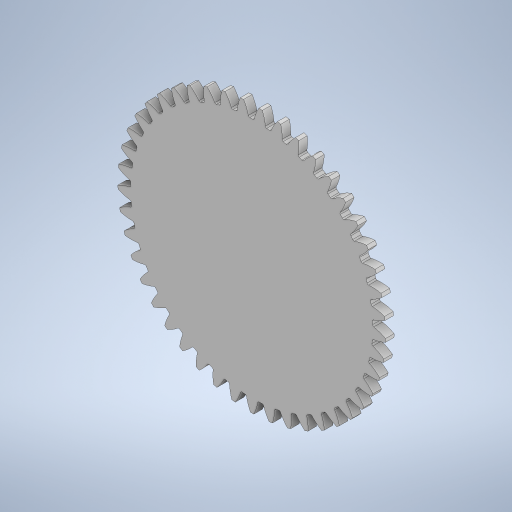
# Autodesk Inventor part: 45G_Recto
Saved by Autodesk Inventor 2023 (Build 270158030, 158C)
## iProperties
Created: 2022-05-28
Part Number: 45G_Recto
Material: Genérico
Document SubType Name: Modeling
Designer: isaac
Density: 1 g/cm^3
Appearance: Valor por defecto
Author: isaac
Autodesk Inventor part; units mm, degrees
ref_plane "YZ Plane" through (0, 0, 0) normal (1, 0, 0) x (0, 1, 0)
ref_plane "XZ Plane" through (0, 0, 0) normal (0, 1, 0) x (-1, 0, 0)
ref_plane "XY Plane" through (0, 0, 0) normal (0, 0, 1) x (1, 0, 0)
sketch "Boceto1" plane through (0, 0, 0) normal (0, 0, 1) x (1, 0, 0)
  arc A0 (469.5392, -20.8063) -> (469.9159, -8.8935) centre (0, 0) ccw
  circle A1 centre (0, 0) radius 425
  arc A2 (469.9159, -8.8935) -> (424.9458, 6.7895) centre (397.36, -144.6272) ccw
  arc A3 (423.6683, -33.6175) -> (469.5392, -20.8063) centre (405.7018, 119.2394) ccw
  arc A4 (467.8654, 44.7434) -> (466.5804, 56.5927) centre (0, 0) ccw
  arc A5 (466.5804, 56.5927) -> (419.8653, 65.8645) centre (413.6211, -87.9179) ccw
  arc A6 (424.2239, 25.6729) -> (467.8654, 44.7434) centre (385.1587, 174.5417) ccw
  arc A7 (457.0851, 109.4223) -> (454.1635, 120.9774) centre (0, 0) ccw
  arc A8 (454.1635, 120.9774) -> (406.6126, 123.6574) centre (421.8316, -29.4973) ccw
  arc A9 (416.5224, 84.4636) -> (457.0851, 109.4223) centre (357.1188, 226.4468) ccw
  arc A10 (437.4081, 171.9713) -> (432.9068, 183.0074) centre (0, 0) ccw
  arc A11 (432.9068, 183.0074) -> (385.4457, 179.0435) centre (421.8316, 29.4973) ccw
  arc A12 (400.7137, 141.6104) -> (437.4081, 171.9713) centre (322.1281, 273.9444) ccw
  arc A13 (409.2175, 231.1731) -> (403.2241, 241.4754) centre (0, 0) ccw
  arc A14 (403.2241, 241.4754) -> (356.7766, 230.9448) centre (413.6211, 87.9179) ccw
  arc A15 (377.1057, 196.0008) -> (409.2175, 231.1731) centre (280.8674, 316.1099) ccw
  arc A16 (373.062, 285.8755) -> (365.693, 295.2433) centre (0, 0) ccw
  arc A17 (365.693, 295.2433) -> (321.1631, 278.3509) centre (397.36, 144.6272) ccw
  arc A18 (346.1577, 246.5763) -> (373.062, 285.8755) centre (234.1401, 352.1228) ccw
  arc A19 (329.6452, 335.0135) -> (321.0442, 343.2646) centre (0, 0) ccw
  arc A20 (321.0442, 343.2646) -> (279.2986, 320.3393) centre (373.3647, 198.5215) ccw
  arc A21 (308.4721, 292.3525) -> (329.6452, 335.0135) centre (182.8554, 381.2819) ccw
  arc A22 (279.8122, 377.6309) -> (270.1466, 384.6047) centre (0, 0) ccw
  arc A23 (270.1466, 384.6047) -> (231.9979, 356.0927) centre (342.1023, 248.5519) ccw
  arc A24 (264.7825, 332.4383) -> (279.8122, 377.6309) centre (128.0117, 403.0199) ccw
  arc A25 (224.533, 412.8982) -> (213.9909, 418.4589) centre (0, 0) ccw
  arc A26 (213.9909, 418.4589) -> (180.1816, 384.9151) centre (304.1812, 293.7444) ccw
  arc A27 (215.9391, 366.0537) -> (224.533, 412.8982) centre (70.6764, 416.9135) ccw
  arc A28 (164.8836, 440.1289) -> (153.6702, 444.1683) centre (0, 0) ccw
  arc A29 (153.6702, 444.1683) -> (124.8582, 406.2455) centre (260.3396, 333.2196) ccw
  arc A30 (162.8928, 392.5442) -> (164.8836, 440.1289) centre (11.9654, 422.6924) ccw
  arc A31 (102.0248, 458.7929) -> (90.3584, 461.2324) centre (0, 0) ccw
  arc A32 (90.3584, 461.2324) -> (67.1047, 419.6689) centre (211.4308, 366.209) ccw
  arc A33 (106.676, 411.3943) -> (102.0248, 458.7929) centre (-46.9785, 420.244) ccw
  arc A34 (37.1803, 468.5271) -> (25.2879, 469.3192) centre (0, 0) ccw
  arc A35 (25.2879, 469.3192) -> (8.045, 424.9238) centre (158.4068, 392.0705) ccw
  arc A36 (48.3828, 422.237) -> (37.1803, 468.5271) centre (-105.0079, 409.6161) ccw
  arc A37 (-28.3879, 469.1419) -> (-40.2748, 468.2712) centre (0, 0) ccw
  arc A38 (-40.2748, 468.2712) -> (-51.1713, 421.9082) centre (102.2995, 410.3009) ccw
  arc A39 (-10.8521, 424.8614) -> (-28.3879, 469.1419) centre (-160.9935, 391.0154) ccw
  arc A40 (-93.4036, 460.6254) -> (-105.0536, 458.1089) centre (0, 0) ccw
  arc A41 (-105.0536, 458.1089) -> (-109.3915, 410.6805) centre (44.2011, 420.5452) ccw
  arc A42 (-69.8758, 419.2164) -> (-93.4036, 460.6254) centre (-213.8456, 364.8041) ccw
  arc A43 (-156.6012, 443.1434) -> (-167.7877, 439.0299) centre (0, 0) ccw
  arc A44 (-167.7877, 439.0299) -> (-165.4826, 391.4595) centre (-14.7577, 422.6041) ccw
  arc A45 (-127.5394, 405.4118) -> (-156.6012, 443.1434) centre (-262.5354, 331.4923) ccw
  arc A46 (-216.7508, 417.0361) -> (-227.256, 411.4058) centre (0, 0) ccw
  arc A47 (-227.256, 411.4058) -> (-218.3528, 364.6191) centre (-73.4292, 416.4375) ccw
  arc A48 (-182.7206, 383.7163) -> (-216.7508, 417.0361) centre (-306.1152, 291.7284) ccw
  arc A49 (-272.6816, 382.8116) -> (-282.3009, 375.7741) centre (0, 0) ccw
  arc A50 (-282.3009, 375.7741) -> (-266.9729, 330.6818) centre (-130.6714, 402.1654) ccw
  arc A51 (-234.3454, 354.5522) -> (-272.6816, 382.8116) centre (-343.7369, 246.2863) ccw
  arc A52 (-323.305, 341.1362) -> (-331.8513, 332.8284) centre (0, 0) ccw
  arc A53 (-331.8513, 332.8284) -> (-310.3968, 290.3082) centre (-185.3704, 380.0656) ccw
  arc A54 (-281.4089, 318.4871) -> (-323.305, 341.1362) centre (-374.6681, 196.0506) ccw
  arc A55 (-367.6356, 292.8209) -> (-374.9425, 283.4046) centre (0, 0) ccw
  arc A56 (-374.9425, 283.4046) -> (-347.7791, 244.284) centre (-236.4613, 350.5682) ccw
  arc A57 (-322.995, 276.2231) -> (-367.6356, 292.8209) centre (-398.3068, 141.9989) ccw
  arc A58 (-404.8106, 238.8062) -> (-410.7358, 228.4646) centre (0, 0) ccw
  arc A59 (-410.7358, 228.4646) -> (-378.3923, 193.5052) centre (-282.9497, 314.2475) ccw
  arc A60 (-358.2945, 228.5827) -> (-404.8106, 238.8062) centre (-414.1929, 85.1834) ccw
  arc A61 (-434.1064, 180.1434) -> (-438.5347, 169.0778) centre (0, 0) ccw
  arc A62 (-438.5347, 169.0778) -> (-401.6406, 138.96) centre (-323.9308, 271.8102) ccw
  arc A63 (-386.6202, 176.4932) -> (-434.1064, 180.1434) centre (-422.0173, 26.7099) ccw
  arc A64 (-454.9528, 117.9743) -> (-457.798, 106.4001) centre (0, 0) ccw
  arc A65 (-457.798, 106.4001) -> (-417.0713, 81.71) centre (-358.607, 224.0825) ccw
  arc A66 (-407.4207, 120.9684) -> (-454.9528, 117.9743) centre (-421.6275, -32.2835) ccw
  arc A67 (-466.9441, 53.509) -> (-468.1508, 41.6515) centre (0, 0) ccw
  arc A68 (-468.1508, 41.6515) -> (-424.3842, 22.8697) centre (-386.3034, 171.9933) ccw
  arc A69 (-420.2913, 63.0892) -> (-466.9441, 53.509) centre (-413.0313, -90.6486) ccw
  arc A70 (-469.8468, -11.9978) -> (-469.3915, -23.9079) centre (0, 0) ccw
  arc A71 (-469.3915, -23.9079) -> (-423.437, -36.4157) centre (-406.4807, 116.5565) ccw
  arc A72 (-424.9813, 3.982) -> (-469.8468, -11.9978) centre (-396.3958, -147.2492) ccw
  arc A73 (-463.6046, -77.2711) -> (-461.4961, -89.0019) centre (0, 0) ccw
  arc A74 (-461.4961, -89.0019) -> (-414.2481, -94.9923) centre (-418.7464, 58.851) ccw
  arc A75 (-421.3996, -55.2028) -> (-463.6046, -77.2711) centre (-372.045, -200.9838) ccw
  arc A76 (-448.3387, -141.0404) -> (-444.6182, -152.3636) centre (0, 0) ccw
  arc A77 (-444.6182, -152.3636) -> (-396.9962, -151.7201) centre (-422.8617, 0) ccw
  arc A78 (-409.6159, -113.313) -> (-448.3387, -141.0404) centre (-340.4528, -250.8065) ccw
  arc A79 (-424.3465, -202.0644) -> (-419.0863, -212.7597) centre (0, 0) ccw
  arc A80 (-419.0863, -212.7597) -> (-372.0174, -205.4947) centre (-418.7464, -58.851) ccw
  arc A81 (-389.8594, -169.2178) -> (-424.3465, -202.0644) centre (-302.234, -295.7476) ccw
  arc A82 (-392.0949, -259.1556) -> (-385.3974, -269.0146) centre (0, 0) ccw
  arc A83 (-385.3974, -269.0146) -> (-339.7976, -255.2697) centre (-406.4807, -116.5565) ccw
  arc A84 (-362.5147, -221.8289) -> (-392.0949, -259.1556) centre (-258.1325, -334.9322) ccw
  arc A85 (-352.2115, -311.2026) -> (-344.2071, -320.0336) centre (0, 0) ccw
  arc A86 (-344.2071, -320.0336) -> (-300.964, -300.0761) centre (-386.3034, -171.9933) ccw
  arc A87 (-328.1142, -270.1224) -> (-352.2115, -311.2026) centre (-209.0069, -367.5978) ccw
  arc A88 (-305.4728, -357.1923) -> (-296.3172, -364.8234) centre (0, 0) ccw
  arc A89 (-296.3172, -364.8234) -> (-256.2725, -339.0419) centre (-358.607, -224.0825) ccw
  arc A90 (-287.3272, -313.1582) -> (-305.4728, -357.1923) centre (-155.8131, -393.1085) ccw
  arc A91 (-252.7884, -396.2298) -> (-242.6599, -402.5123) centre (0, 0) ccw
  arc A92 (-242.6599, -402.5123) -> (-206.593, -371.4086) centre (-323.9308, -271.8102) ccw
  arc A93 (-240.9477, -350.0988) -> (-252.7884, -396.2298) centre (-99.5866, -410.9678) ccw
  arc A94 (-195.1838, -427.555) -> (-184.2795, -432.3668) centre (0, 0) ccw
  arc A95 (-184.2795, -432.3668) -> (-152.8924, -396.5462) centre (-282.9497, -314.2475) ccw
  arc A96 (-189.8785, -380.2251) -> (-195.1838, -427.555) centre (-41.4218, -420.828) ccw
  arc A97 (-133.7801, -450.5584) -> (-122.3122, -453.8058) centre (0, 0) ccw
  arc A98 (-122.3122, -453.8058) -> (-96.2158, -413.9656) centre (-236.4613, -350.5682) ccw
  arc A99 (-135.1135, -402.9508) -> (-133.7801, -450.5584) centre (17.5493, -422.4974) ccw
  arc A100 (-69.7725, -464.7922) -> (-57.9643, -466.412) centre (0, 0) ccw
  arc A101 (-57.9643, -466.412) -> (-37.6666, -423.3276) centre (-185.3704, -380.0656) ccw
  arc A102 (-77.7187, -417.8335) -> (-69.7725, -464.7922) centre (76.1788, -415.9433) ccw
  arc A103 (-4.4069, -469.9793) -> (7.5118, -469.94) centre (0, 0) ccw
  arc A104 (7.5118, -469.94) -> (21.6158, -424.4499) centre (-130.6714, -402.1654) ccw
  arc A105 (-18.8112, -424.5835) -> (-4.4069, -469.9793) centre (133.3255, -401.2933) ccw
  arc A106 (61.0444, -466.0189) -> (72.8417, -464.3211) centre (0, 0) ccw
  arc A107 (72.8417, -464.3211) -> (80.4774, -417.3109) centre (-73.4292, -416.4375) ccw
  arc A108 (40.4625, -423.0695) -> (61.0444, -466.0189) centre (187.8772, -378.8326) ccw
  arc A109 (125.3076, -452.9879) -> (136.7538, -449.6648) centre (0, 0) ccw
  arc A110 (136.7538, -449.6648) -> (137.7727, -402.0494) centre (-14.7577, -422.6041) ccw
  arc A111 (98.9486, -413.3209) -> (125.3076, -452.9879) centre (238.7721, -348.9984) ccw
  arc A112 (187.1319, -431.14) -> (198.0042, -426.2562) centre (0, 0) ccw
  arc A113 (198.0042, -426.2562) -> (192.3863, -378.9624) centre (44.2011, -420.5452) ccw
  arc A114 (155.5088, -395.5275) -> (187.1319, -431.14) centre (285.0196, -312.3713) ccw
  arc A115 (245.3138, -400.9004) -> (255.4006, -394.5511) centre (0, 0) ccw
  arc A116 (255.4006, -394.5511) -> (243.2554, -348.4994) centre (102.2995, -410.3009) ccw
  arc A117 (209.0422, -370.0356) -> (245.3138, -400.9004) centre (325.7195, -269.6643) ccw
  arc A118 (298.721, -362.8578) -> (307.8259, -355.1664) centre (0, 0) ccw
  arc A119 (307.8259, -355.1664) -> (289.3898, -311.2532) centre (158.4068, -392.0705) ccw
  arc A120 (258.5068, -337.3414) -> (298.721, -362.8578) centre (360.0796, -221.7085) ccw
  arc A121 (346.3139, -317.7526) -> (354.2598, -308.8689) centre (0, 0) ccw
  arc A122 (354.2598, -308.8689) -> (329.8916, -267.9488) centre (211.4308, -366.209) ccw
  arc A123 (302.9399, -298.0812) -> (346.3139, -317.7526) centre (387.4312, -169.4375) ccw
  arc A124 (387.1662, -266.4626) -> (393.7984, -256.5596) centre (0, 0) ccw
  arc A125 (393.7984, -256.5596) -> (363.9723, -219.4291) centre (260.3396, -333.2196) ccw
  arc A126 (341.4766, -253.0192) -> (387.1662, -266.4626) centre (407.2419, -113.8685) ccw
  arc A127 (420.4828, -209.9863) -> (425.6722, -199.2566) centre (0, 0) ccw
  arc A128 (425.6722, -199.2566) -> (390.9688, -166.6385) centre (304.1812, -293.7444) ccw
  arc A129 (373.3668, -203.0325) -> (420.4828, -209.9863) centre (419.1261, -56.0832) ccw
  arc A130 (445.6151, -149.4229) -> (449.2607, -138.0753) centre (0, 0) ccw
  arc A131 (449.2607, -138.0753) -> (410.3555, -110.6044) centre (342.1023, -248.5519) ccw
  arc A132 (397.9899, -149.094) -> (445.6151, -149.4229) centre (422.8525, 2.7936) ccw
  arc A133 (462.074, -85.951) -> (464.1049, -74.2066) centre (0, 0) ccw
  arc A134 (464.1049, -74.2066) -> (421.7551, -52.4176) centre (373.3647, -198.5215) ccw
  arc A135 (414.8666, -92.2535) -> (462.074, -85.951) centre (418.3485, 61.6161) ccw
  point P0 (424.2239, 25.6729)
  point P1 (419.8653, 65.8645)
  point P2 (416.5224, 84.4636)
  point P3 (406.6126, 123.6574)
  point P4 (400.7137, 141.6104)
  point P5 (385.4457, 179.0435)
  point P6 (377.1057, 196.0008)
  point P7 (356.7766, 230.9448)
  point P8 (346.1577, 246.5763)
  point P9 (308.4721, 292.3525)
  point P10 (279.2986, 320.3393)
  point P11 (264.7825, 332.4383)
  point P12 (231.9979, 356.0927)
  point P13 (215.9391, 366.0537)
  point P14 (180.1816, 384.9151)
  point P15 (162.8928, 392.5442)
  point P16 (124.8582, 406.2455)
  point P17 (106.676, 411.3943)
  point P18 (67.1047, 419.6689)
  point P19 (48.3828, 422.237)
  point P20 (8.045, 424.9238)
  point P21 (-10.8521, 424.8614)
  point P22 (-51.1713, 421.9082)
  point P23 (-69.8758, 419.2164)
  point P24 (-109.3915, 410.6805)
  point P25 (-127.5394, 405.4118)
  point P26 (-165.4826, 391.4595)
  point P27 (-182.7206, 383.7163)
  point P28 (-218.3528, 364.6191)
  point P29 (-234.3454, 354.5522)
  point P30 (-266.9729, 330.6818)
  point P31 (-281.4089, 318.4871)
  point P32 (-310.3968, 290.3082)
  point P33 (-322.995, 276.2231)
  point P34 (-347.7791, 244.284)
  point P35 (-358.2945, 228.5827)
  point P36 (-386.6202, 176.4932)
  point P37 (-401.6406, 138.96)
  point P38 (-407.4207, 120.9684)
  point P39 (-420.2913, 63.0892)
  point P40 (-424.3842, 22.8697)
  point P41 (-424.9813, 3.982)
  point P42 (-423.437, -36.4157)
  point P43 (-421.3996, -55.2028)
  point P44 (-409.6159, -113.313)
  point P45 (-396.9962, -151.7201)
  point P46 (-389.8594, -169.2178)
  point P47 (-372.0174, -205.4947)
  point P48 (-362.5147, -221.8289)
  point P49 (-339.7976, -255.2697)
  point P50 (-328.1142, -270.1224)
  point P51 (-300.964, -300.0761)
  point P52 (-287.3272, -313.1582)
  point P53 (-240.9477, -350.0988)
  point P54 (-206.593, -371.4086)
  point P55 (-189.8785, -380.2251)
  point P56 (-152.8924, -396.5462)
  point P57 (-135.1135, -402.9508)
  point P58 (-96.2158, -413.9656)
  point P59 (-77.7187, -417.8335)
  point P60 (-37.6666, -423.3276)
  point P61 (-18.8112, -424.5835)
  point P62 (40.4625, -423.0695)
  point P63 (98.9486, -413.3209)
  point P64 (137.7727, -402.0494)
  point P65 (155.5088, -395.5275)
  point P66 (192.3863, -378.9624)
  point P67 (209.0422, -370.0356)
  point P68 (243.2554, -348.4994)
  point P69 (258.5068, -337.3414)
  point P70 (289.3898, -311.2532)
  point P71 (302.9399, -298.0812)
  point P72 (329.8916, -267.9488)
  point P73 (341.4766, -253.0192)
  point P74 (363.9723, -219.4291)
  point P75 (373.3668, -203.0325)
  point P76 (390.9688, -166.6385)
  point P77 (397.9899, -149.094)
  point P78 (410.3555, -110.6044)
  point P79 (414.8666, -92.2535)
  point P80 (421.7551, -52.4176)
  point P81 (423.6683, -33.6175)
  dimension "d8" = 360
  constraints: 270 point on circle, 135 centre point, 3 coincident, 451 other
extrude "Extrusión1" add sketch "Boceto1" along normal blind 30
fillet "Empalme1" radius 5.235 2 edges at (264.7825, 332.4383, 15) (279.2986, 320.3393, 15)
pattern_circular "Patrón circular1" count 45 over 360 about axis through (0, 0, 0) along (0, 0, 1) of "Empalme1"
